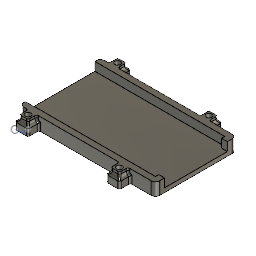
Base_96 (Autodesk Fusion 360 design; units mm, degrees)
Autodesk Fusion 360 part; units mm, degrees
sketch "Sketch1" plane through (0, 0, 0) normal (0, 0, 1) x (1, 0, 0)
  line L0 (-68.38, 47.37) -> (68.38, 47.37)
  line L1 (68.38, 47.37) -> (68.38, -47.37)
  line L2 (68.38, -47.37) -> (-68.38, -47.37)
  line L3 (-68.38, -47.37) -> (-68.38, 47.37)
  line L4 (-68.38, 47.37) -> (68.38, -47.37) construction
  line L5 (68.38, 47.37) -> (-68.38, -47.37) construction
  line L6 (-58.38, 57.37) -> (-48.38, 57.37)
  line L7 (-48.38, 57.37) -> (-48.38, 47.37)
  line L8 (-48.38, 47.37) -> (-58.38, 47.37)
  line L9 (-58.38, 47.37) -> (-58.38, 57.37)
  line L10 (48.38, 57.37) -> (58.38, 57.37)
  line L11 (58.38, 57.37) -> (58.38, 47.37)
  line L12 (58.38, 47.37) -> (48.38, 47.37)
  line L13 (48.38, 47.37) -> (48.38, 57.37)
  line L14 (48.38, -47.37) -> (58.38, -47.37)
  line L15 (58.38, -47.37) -> (58.38, -57.37)
  line L16 (58.38, -57.37) -> (48.38, -57.37)
  line L17 (48.38, -57.37) -> (48.38, -47.37)
  line L18 (-58.38, -47.37) -> (-48.38, -47.37)
  line L19 (-48.38, -47.37) -> (-48.38, -57.37)
  line L20 (-48.38, -57.37) -> (-58.38, -57.37)
  line L21 (-58.38, -57.37) -> (-58.38, -47.37)
  point P0 (-57.3369, -42.2056)
  point P1 (-53.88, -84.89)
  dimension "d1" = 136.76
  dimension "d2" = 94.74
  dimension "d3" = 10
  dimension "d4" = 10
  dimension "d5" = 10
  dimension "d6" = 10
  constraint perpendicular L0 L1
  constraint parallel L0 L2
  constraint parallel L1 L3
  constraint horizontal L0
  constraint horizontal L6
  constraint vertical L7
  constraint horizontal L8
  constraint vertical L9
  constraint coincident L0 L7.end
  constraint horizontal L10
  constraint vertical L11
  constraint horizontal L12
  constraint vertical L13
  constraint horizontal L14
  constraint vertical L15
  constraint horizontal L16
  constraint vertical L17
  constraint horizontal L18
  constraint vertical L19
  constraint horizontal L20
  constraint vertical L21
  measures "d1" distance of L1 L3
  measures "d2" distance of L0.start L2.end
  measures "d3" distance of L6.start L6.end
  measures "d4" distance of L6.start L8.end
  measures "d5" distance of L10.start L10.end
  measures "d6" distance of L10.start L12.end
  measures "d79" distance of L0.end
extrude "Extrude1" add sketch "Sketch1" along normal blind 15
ref_plane "WorkPlane1" through (0, 0, 15) normal (0, 0, 1) x (1, 0, 0)
sketch "Sketch2" plane through (0, 0, 15) normal (0, 0, 1) x (1, 0, 0)
  line L0 (68.38, -40.5) -> (-68.38, -40.5)
  line L1 (-68.38, -40.5) -> (-68.38, 40.5)
  line L2 (-68.38, 40.5) -> (68.38, 40.5)
  line L3 (68.38, 40.5) -> (68.38, -40.5)
  line L4 (68.38, -40.5) -> (-68.38, 40.5) construction
  line L5 (-68.38, -40.5) -> (68.38, 40.5) construction
  dimension "d18" = 136.76
  dimension "d19" = 81
  constraint perpendicular L0 L1
  constraint parallel L0 L2
  constraint parallel L1 L3
  constraint horizontal L0
  constraint coincident L4 origin
  constraint coincident L5 origin
  measures "d18" distance of L1.end L2.end
  measures "d19" distance of L0.end L1.end
extrude "Extrude2" cut sketch "Sketch2" against normal blind 10
ref_plane "WorkPlane2" through (68.38, 0, 7.5) normal (1, 0, 0) x (0, 1, 0)
sketch "Sketch3" plane through (68.38, 0, 7.5) normal (1, 0, 0) x (0, 1, 0)
  line L0 (42, -7.5) -> (-42, -7.5)
  line L1 (-42, -7.5) -> (-42, 7.5)
  line L2 (-42, 7.5) -> (42, 7.5)
  line L3 (42, 7.5) -> (42, -7.5)
  line L4 (42, -7.5) -> (-42, 7.5) construction
  line L5 (-42, -7.5) -> (42, 7.5) construction
  dimension "d23" = 84
  dimension "d24" = 15
  constraint perpendicular L0 L1
  constraint parallel L0 L2
  constraint parallel L1 L3
  constraint horizontal L0
  constraint coincident L4 origin
  constraint coincident L5 origin
  measures "d23" distance of L1.end L2.end
  measures "d24" distance of L0.end L1.end
sketch "Sketch5" plane through (7.88, 0, 15) normal (0, 0, 1) x (1, 0, 0)
  circle A0 centre (-61.26, 52.37) radius 3.25
  circle A1 centre (45.5, 52.37) radius 3.25
  circle A2 centre (-61.26, -52.37) radius 3.25
  circle A3 centre (45.5, -52.37) radius 3.25
  dimension "d29" = 6.5
  dimension "d32" = 106.76
  dimension "d33" = -104.74
  measures "d29" diameter of A0
extrude "Extrude4" cut sketch "Sketch5" against normal blind 15
ref_plane "WorkPlane7" through (68.38, 0, 7.5) normal (1, 0, 0) x (0, 1, 0)
sketch "Sketch8" plane through (68.38, 0, 7.5) normal (1, 0, 0) x (0, 1, 0)
  line L0 (0, -7.5) -> (-42, -7.5)
  line L1 (-42, -7.5) -> (42, -7.5)
  line L2 (42, -7.5) -> (42, 7.5)
  line L3 (42, 7.5) -> (-42, 7.5)
  line L4 (-42, 7.5) -> (-42, -7.5)
  dimension "d52" = 42
  dimension "d53" = 84
  dimension "d54" = 15
  constraint horizontal L0
  constraint horizontal L1
  constraint vertical L2
  constraint horizontal L3
  constraint vertical L4
  measures "d52" distance of L0.start L0.end
  measures "d53" distance of L0.end L1.end
  measures "d54" distance of L0.end L3.end
ref_plane "WorkPlane12" through (68.38, 0, 7.5) normal (1, 0, 0) x (0, 1, 0)
sketch "Sketch13" plane through (68.38, 0, 7.5) normal (1, 0, 0) x (0, 1, 0)
  line L0 (47.37, -22.5) -> (-47.37, -22.5)
  line L1 (-47.37, -22.5) -> (-47.37, 7.5)
  line L2 (-47.37, 7.5) -> (47.37, 7.5)
  line L3 (47.37, 7.5) -> (47.37, -22.5)
  line L4 (47.37, -22.5) -> (-47.37, 7.5) construction
  line L5 (-47.37, -22.5) -> (47.37, 7.5) construction
  line L6 (-47.37, -7.5) -> (47.37, -7.5)
  point P0 (0, -7.5)
  dimension "d78" = 94.74
  dimension "d79" = 30
  constraint perpendicular L0 L1
  constraint parallel L0 L2
  constraint parallel L1 L3
  constraint horizontal L0
  constraint coincident L4 P0
  constraint coincident L5 P0
  constraint midpoint L1 L6.start
  constraint midpoint L3 L6.end
  measures "d78" distance of L1.end L2.end
  measures "d79" distance of L0.end L1.end
extrude "Extrude10" add sketch "Sketch13" along normal blind 22.07 contours L1 L2 L3 L6
ref_plane "WorkPlane13" through (90.45, 0, 7.5) normal (1, 0, 0) x (0, 0, -1)
ref_plane "WorkPlane15" through (68.38, 0, 10) normal (-1, 0, 0) x (0, -1, 0)
sketch "Sketch17" plane through (68.38, 0, 0) normal (-1, 0, 0) x (0, -1, 0)
  line L0 (40.5, 5) -> (40.5, 15)
  line L1 (40.5, 15) -> (-40.5, 15)
  line L2 (-40.5, 15) -> (-40.5, 5)
  line L3 (-40.5, 5) -> (40.5, 5)
  line L4 (40.5, 5) -> (-40.5, 5)
  line L5 (-40.5, 5) -> (-40.5, 25)
  line L6 (-40.5, 25) -> (40.5, 25)
  line L7 (40.5, 25) -> (40.5, 5)
  line L8 (40.5, 5) -> (-40.5, 25) construction
  line L9 (-40.5, 5) -> (40.5, 25) construction
  point P0 (0, 15)
  dimension "d93" = 81
  dimension "d94" = 20
  constraint perpendicular L4 L5
  constraint parallel L4 L6
  constraint parallel L5 L7
  constraint horizontal L4
  constraint coincident L8 P0
  constraint coincident L9 P0
  constraint midpoint L1 P0
  measures "d93" distance of L5.end L6.end
  measures "d94" distance of L2.end L5.end
extrude "Extrude13" cut sketch "Sketch17" against normal blind 15.2 contours L0 L1 L2 L3 L4 L5 L7
sketch "Sketch14" plane through (90.45, 0, 7.5) normal (1, 0, 0) x (0, 1, 0)
  line L0 (36.75, -2.5) -> (-36.75, -2.5)
  line L1 (-36.75, -2.5) -> (-36.75, 17.5)
  line L2 (-36.75, 17.5) -> (36.75, 17.5)
  line L3 (36.75, 17.5) -> (36.75, -2.5)
  line L4 (36.75, -2.5) -> (-36.75, 17.5) construction
  line L5 (-36.75, -2.5) -> (36.75, 17.5) construction
  line L6 (-36.75, 7.5) -> (36.75, 7.5)
  point P0 (0, 7.5)
  dimension "d83" = 73.5
  dimension "d84" = 20
  constraint perpendicular L0 L1
  constraint parallel L0 L2
  constraint parallel L1 L3
  constraint horizontal L0
  constraint coincident L4 P0
  constraint coincident L5 P0
  constraint midpoint L1 L6.start
  constraint midpoint L3 L6.end
  measures "d83" distance of L1.end L2.end
  measures "d84" distance of L0.end L1.end
extrude "Extrude11" cut sketch "Sketch14" against normal blind 32.07 contours L0 L1 L3 L6
fillet "Fillet9" radius 5 4 edges at (-68.38, -47.37, 7.5) (90.45, -47.37, 7.5) (90.45, 47.37, 7.5) (-68.38, 47.37, 7.5)
ref_plane "WorkPlane16" through (0, 0, 0) normal (0, 0, 1) x (1, 0, 0)
sketch "Sketch18" plane through (0, 0, 0) normal (0, 0, 1) x (1, 0, 0)
  line L0 (-58.38, -57.37) -> (-53.38, -57.37)
  line L1 (-53.38, -57.37) -> (-53.38, -52.37)
  line L2 (-45.63, -60.12) -> (-61.13, -60.12)
  line L3 (-61.13, -60.12) -> (-61.13, -44.62)
  line L4 (-61.13, -44.62) -> (-45.63, -44.62)
  line L5 (-45.63, -44.62) -> (-45.63, -60.12)
  line L6 (-45.63, -60.12) -> (-61.13, -44.62) construction
  line L7 (-61.13, -60.12) -> (-45.63, -44.62) construction
  line L8 (45.63, -44.62) -> (61.13, -44.62)
  line L9 (45.63, -60.12) -> (45.63, -44.62)
  line L10 (61.13, -60.12) -> (45.63, -60.12)
  line L11 (61.13, -44.62) -> (61.13, -60.12)
  line L12 (-61.13, 60.12) -> (-45.63, 60.12)
  line L13 (-61.13, 44.62) -> (-61.13, 60.12)
  line L14 (-45.63, 44.62) -> (-61.13, 44.62)
  line L15 (-45.63, 60.12) -> (-45.63, 44.62)
  line L16 (45.63, 60.12) -> (61.13, 60.12)
  line L17 (45.63, 44.62) -> (45.63, 60.12)
  line L18 (61.13, 44.62) -> (45.63, 44.62)
  line L19 (61.13, 60.12) -> (61.13, 44.62)
  point P0 (-53.38, -52.37)
  dimension "d99" = 5
  dimension "d100" = 5
  dimension "d101" = 15.5
  dimension "d102" = 15.5
  dimension "d105" = 106.76
  dimension "d106" = 104.74
  constraint horizontal L0
  constraint perpendicular L0 L1
  constraint perpendicular L2 L3
  constraint parallel L2 L4
  constraint parallel L3 L5
  constraint horizontal L2
  constraint coincident L6 P0
  constraint coincident L7 P0
  constraint coincident P0 L1.end
  measures "d99" distance of L0.start L0.end
  measures "d100" distance of L0.end P0
  measures "d101" distance of L3.end L4.end
  measures "d102" distance of L2.end L3.end
extrude "Extrude14" add sketch "Sketch18" along normal blind 8
fillet "Fillet10" radius 5 12 edges at (48.38, -52.37, 8) (53.38, -57.37, 8) (58.38, -52.37, 8) (-48.38, -52.37, 8) (-53.38, -57.37, 8) (-58.38, -52.37, 8) (-58.38, 52.37, 8) (-53.38, 57.37, 8) (48.38, 52.37, 8) (53.38, 57.37, 8) (-48.38, 52.37, 8) (58.38, 52.37, 8)
extrude "Extrude15" cut 4 faces at (-55.2454, -51.4717, 8) (-55.2454, 53.2683, 8) (51.5146, 53.2683, 8) (51.5146, -51.4717, 8) along direction (0, 0, -1) blind 8
ref_plane "WorkPlane17" through (0, 0, 0) normal (0, 0, 1) x (1, 0, 0)
sketch "Sketch19" plane through (0, 0, 0) normal (0, 0, 1) x (1, 0, 0)
  line L0 (-61, -60) -> (-53.4, -60)
  line L1 (-53.4, -60) -> (-53.4, -52.4)
  dimension "d120" = 7.6
  dimension "d121" = 7.6
  constraint horizontal L0
  constraint perpendicular L0 L1
  measures "d120" distance of L0.start L0.end
  measures "d121" distance of L0.end L1.end
ref_plane "WorkPlane18" through (0, 0, 0) normal (0, 0, 1) x (1, 0, 0)
sketch "Sketch20" plane through (0, 0, 0) normal (0, 0, 1) x (1, 0, 0)
  line L0 (61.13, 60.12) -> (53.38, 60.12)
  line L1 (53.38, 60.12) -> (53.38, 52.37)
  line L2 (47.9798, 49.2235) -> (53.4049, 46.1201)
  line L3 (53.4049, 46.1201) -> (58.805, 49.2666)
  line L4 (58.805, 49.2666) -> (58.7802, 55.5165)
  line L5 (58.7802, 55.5165) -> (53.3551, 58.62)
  line L6 (53.3551, 58.62) -> (47.955, 55.4734)
  line L7 (47.955, 55.4734) -> (47.9798, 49.2235)
  line L8 (-58.805, 55.4734) -> (-58.7802, 49.2235)
  line L9 (-58.7802, 49.2235) -> (-53.3551, 46.1201)
  line L10 (-53.4049, 58.62) -> (-58.805, 55.4734)
  line L11 (-47.9798, 55.5165) -> (-53.4049, 58.62)
  line L12 (-53.3551, 46.1201) -> (-47.955, 49.2666)
  line L13 (-47.955, 49.2666) -> (-47.9798, 55.5165)
  line L14 (47.955, -49.2666) -> (47.9798, -55.5165)
  line L15 (47.9798, -55.5165) -> (53.4049, -58.6199)
  line L16 (53.3551, -46.12) -> (47.955, -49.2666)
  line L17 (58.7802, -49.2235) -> (53.3551, -46.12)
  line L18 (53.4049, -58.6199) -> (58.805, -55.4734)
  line L19 (58.805, -55.4734) -> (58.7802, -49.2235)
  line L20 (-58.805, -49.2666) -> (-58.7802, -55.5165)
  line L21 (-58.7802, -55.5165) -> (-53.3551, -58.6199)
  line L22 (-53.4049, -46.12) -> (-58.805, -49.2666)
  line L23 (-47.9798, -49.2235) -> (-53.4049, -46.12)
  line L24 (-53.3551, -58.6199) -> (-47.955, -55.4734)
  line L25 (-47.955, -55.4734) -> (-47.9798, -49.2235)
  point P0 (53.38, 52.37)
  point P1 (-53.38, 52.37)
  point P2 (-53.38, 52.37)
  point P3 (53.38, -52.37)
  point P4 (53.38, -52.37)
  point P5 (-53.38, -52.37)
  point P6 (-53.38, -52.37)
  dimension "d123" = 7.75
  dimension "d124" = 7.75
  dimension "d125" = 6.25
  dimension "d128" = -106.76
  dimension "d129" = -104.74
  constraint horizontal L0
  constraint perpendicular L0 L1
  constraint coincident P0 L1.end
  measures "d123" distance of L0.start L0.end
  measures "d124" distance of L0.end P0
  measures "d125" distance of L2.start P0
extrude "Extrude16" cut sketch "Sketch20" along normal blind 4
fillet "Fillet11" radius 2 16 edges at (61.13, -47.37, 4) (61.13, -60.12, 4) (45.63, -60.12, 4) (45.63, -47.37, 4) (-45.63, -47.37, 4) (-45.63, -60.12, 4) (-61.13, -47.37, 4) (-61.13, -60.12, 4) (61.13, 47.37, 4) (61.13, 60.12, 4) (45.63, 60.12, 4) (45.63, 47.37, 4) (-61.13, 47.37, 4) (-61.13, 60.12, 4) (-45.63, 60.12, 4) (-45.63, 47.37, 4)
fillet "Fillet13" radius 2 32 edges at (59.0186, 58.0086, 10.0201) (58.38, 57.37, 13.7326) (47.7414, 58.0086, 10.0201) (48.38, 57.37, 13.7326) (47.0028, 47.37, 9.0191) (48.38, 47.37, 13.7326) (-47.7414, 58.0086, 10.0201) (-48.38, 57.37, 13.7326) (-59.0186, 58.0086, 10.0201) (-58.38, 57.37, 13.7326) (-59.7572, 47.37, 9.0191) (-58.38, 47.37, 13.7326) (-59.7572, -47.37, 9.0191) (-58.38, -47.37, 13.7326) (-59.0186, -58.0086, 10.0201) (-58.38, -57.37, 13.7326) (-47.7414, -58.0086, 10.0201) (-48.38, -57.37, 13.7326) (47.0028, -47.37, 9.0191) (48.38, -47.37, 13.7326) (47.7414, -58.0086, 10.0201) (48.38, -57.37, 13.7326) (59.0186, -58.0086, 10.0201) (58.38, -57.37, 13.7326) (-47.0028, -47.37, 9.0191) (-48.38, -47.37, 13.7326) (59.7572, -47.37, 9.0191) (58.38, -47.37, 13.7326) (59.7572, 47.37, 9.0191) (58.38, 47.37, 13.7326) (-47.0028, 47.37, 9.0191) (-48.38, 47.37, 13.7326)
